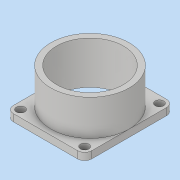
# Autodesk Inventor part: Rohrhalterung
Saved by Autodesk Inventor 2018 (Build 220112000, 112)
## iProperties
Created: 2020-05-25
Part Number: Rohrhalterung
Material: Generisch
Document SubType Name: Modeling
Designer: marce
Density: 1 g/cm^3
Appearance: Vorgabe
Author: marce
Autodesk Inventor part; units mm, degrees
ref_plane "YZ Plane" through (0, 0, 0) normal (1, 0, 0) x (0, 1, 0)
ref_plane "XZ Plane" through (0, 0, 0) normal (0, 1, 0) x (-1, 0, 0)
ref_plane "XY Plane" through (0, 0, 0) normal (0, 0, 1) x (1, 0, 0)
sketch "Skizze1" plane through (0, 0, 0) normal (0, 0, 1) x (1, 0, 0)
  line L0 (-27.5, -31.25) -> (27.5, -31.25)
  line L1 (27.5, -31.25) -> (27.5, 31.25)
  line L2 (27.5, 31.25) -> (-27.5, 31.25)
  line L3 (-27.5, 31.25) -> (-27.5, -31.25)
  point P0 (0, 0)
  point P1 (-27.5, 0)
  point P2 (0, -31.25)
  dimension "d5" = 55
  dimension "d6" = 62.5
  constraints: 8 end point, 2 midpoint, 2 parallel, 1 horizontal, 1 horizontal alignment, 1 perpendicular, 1 vertical alignment
  measures "d5" distance of L2.end L1.end
  measures "d6" distance of L1.end L0.end
extrude "Extrusion1" add sketch "Skizze1" along normal blind 30
sketch "Skizze2" plane through (0, 0, 30) normal (0, 0, 1) x (1, 0, 0)
  line L0 (-22.5, -26.25) -> (22.5, -26.25)
  line L1 (22.5, -26.25) -> (22.5, 26.25)
  line L2 (22.5, 26.25) -> (-22.5, 26.25)
  line L3 (-22.5, 26.25) -> (-22.5, -26.25)
  point P0 (0, 0)
  point P1 (0, 26.25)
  point P2 (-22.5, 0)
  dimension "d3" = 45
  dimension "d4" = 52.5
  constraints: 8 end point, 2 midpoint, 2 parallel, 1 horizontal, 1 horizontal alignment, 1 perpendicular, 1 vertical alignment
  measures "d3" distance of L2.end L1.end
  measures "d4" distance of L1.end L0.end
hole "Bohrung1" at (-22.5, 26.25, 30) at (-22.5, -26.25, 30) at (22.5, -26.25, 30) at (22.5, 26.25, 30) direction (0, 0, -1) diameter 6 end through all
sketch "Skizze3" plane through (0, 0, 30) normal (0, 0, 1) x (1, 0, 0)
  circle A0 centre (0, 0) radius 27.5
  circle A1 centre (22.5, -26.25) radius 3 projected
  circle A2 centre (-22.5, 26.25) radius 3 projected
  circle A3 centre (-22.5, -26.25) radius 3 projected
  circle A4 centre (22.5, 26.25) radius 3 projected
  line L0 (-27.5, -31.25) -> (27.5, -31.25) projected
  line L1 (27.5, -31.25) -> (27.5, 31.25) projected
  line L2 (27.5, 31.25) -> (-27.5, 31.25) projected
  line L3 (-27.5, 31.25) -> (-27.5, -31.25) projected
  dimension "d14" = 55
  constraints: 1 centre point, 1 coincident
  measures "d14" diameter of A0
extrude "Extrusion2" cut sketch "Skizze3" against normal blind 25 contours L1 L0 L3 A0 | A0 L3 L2 L1
sketch "Skizze4" plane through (0, 0, 30) normal (0, 0, 1) x (1, 0, 0)
  circle A0 centre (0, 0) radius 23.5
  dimension "d17" = 47
  constraints: 1 centre point, 1 coincident
  measures "d17" diameter of A0
extrude "Extrusion3" cut sketch "Skizze4" against normal through all
fillet "Rundung1" radius 5 4 edges at (-27.5, -31.25, 2.5) (27.5, -31.25, 2.5) (27.5, 31.25, 2.5) (-27.5, 31.25, 2.5)
